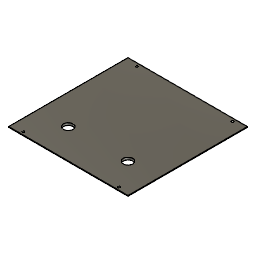
Sol 200x200mm (Autodesk Fusion 360 design; units mm, degrees)
part number: 2026-03-31-14-11-04-905
Autodesk Fusion 360 part; units mm, degrees
sketch "Esquisse1" plane through (0, 0, 0) normal (0, 0, 1) x (1, 0, 0)
  line L0 (0, 0) -> (200, 0)
  line L1 (200, 0) -> (200, 200)
  line L2 (200, 200) -> (0, 200)
  line L3 (0, 200) -> (0, 0)
  dimension "d18" = 200
  dimension "d19" = 200
  constraint horizontal L0
  constraint vertical L1
  constraint horizontal L2
  constraint vertical L3
  constraint coincident L0.start L3.end
  measures "d18" distance of L0 L2
  measures "d19" distance of L1 L3
extrude "Extrusion1" add sketch "Esquisse1" along normal blind 4
chamfer "Chanfrein1" distance 3 angle 45 1 faces at (66.6667, 133.3333, 0)
sketch "Esquisse2" plane through (0, 0, 4) normal (0, 0, 1) x (-1, 0, 0)
  circle A0 centre (-20, -195) radius 2
  circle A1 centre (-180, -195) radius 2
  circle A2 centre (-180, -5) radius 2
  circle A3 centre (-20, -5) radius 2
  line L0 (-20, -5) -> (-20, 0)
  line L1 (-180, -5) -> (-180, 0)
  line L2 (-20, -195) -> (-20, -200)
  line L3 (-180, -195) -> (-180, -200)
  line L4 (-20, -5) -> (0, -5)
  line L5 (-180, -5) -> (-200, -5)
  line L6 (-180, -195) -> (-200, -195)
  line L7 (-20, -195) -> (0, -195)
  line L8 (0, -200) -> (0, 0)
  line L9 (0, 0) -> (-200, 0)
  line L10 (-200, 0) -> (-200, -200)
  line L11 (-200, -200) -> (0, -200)
  dimension "d10" = 4
  dimension "d11" = 4
  dimension "d12" = 4
  dimension "d13" = 4
  dimension "d28" = 5
  dimension "d29" = 5
  dimension "d30" = 5
  dimension "d31" = 5
  dimension "d32" = 20
  dimension "d33" = 20
  dimension "d34" = 20
  dimension "d35" = 20
  constraint coincident A3.centre L0.start
  constraint coincident A2.centre L1.start
  constraint coincident A0.centre L2.start
  constraint coincident A1.centre L3.start
  measures "d10" diameter of A0
  measures "d11" diameter of A1
  measures "d12" diameter of A2
  measures "d13" diameter of A3
  measures "d28" distance of A3.centre L0.end
  measures "d29" distance of A2.centre L1.end
  measures "d30" distance of A0.centre L2.end
  measures "d31" distance of A1.centre L3.end
  measures "d32" distance of A3.centre L4.end
  measures "d33" distance of A2.centre L5.end
  measures "d34" distance of A0.centre L7.end
  measures "d35" distance of A1.centre L6.end
extrude "Extrusion2" cut sketch "Esquisse2" against normal blind 14 contours A0 L2 L7 | A0 L2 L7 | A3 L0 L4 | A3 L0 L4 | A1 L3 L6 | A1 L3 L6 | A2 L1 L5 | A2 L1 L5
thread "Filetage1" "ISO Metric profile 4.0 M4x0.7 M4x0.7 6H" major diameter 4.1095 minor diameter 3.332 pitch 0.7 angle 60 resizes the face on face at (20, 197, 2.6667)
thread "Filetage2" "ISO Metric profile 4.0 M4x0.7 M4x0.7 6H" major diameter 4.1095 minor diameter 3.332 pitch 0.7 angle 60 resizes the face on face at (20, 3, 2.6667)
thread "Filetage3" "ISO Metric profile 4.0 M4x0.7 M4x0.7 6H" major diameter 4.1095 minor diameter 3.332 pitch 0.7 angle 60 resizes the face on face at (180, 3, 2.6667)
thread "Filetage4" "ISO Metric profile 4.0 M4x0.7 M4x0.7 6H" major diameter 4.1095 minor diameter 3.332 pitch 0.7 angle 60 resizes the face on face at (180, 197, 2.6667)
move_face "DécalerLesFaces1" offset -0.05 1 faces at (18.3423, 5.1659, 2.6667)
move_face "DécalerLesFaces2" offset -0.05 1 faces at (180.5306, 6.5792, 2.6667)
move_face "DécalerLesFaces3" offset -0.05 1 faces at (178.3423, 195.1659, 1.3333)
move_face "DécalerLesFaces4" offset -0.05 1 faces at (18.3423, 195.1659, 2.6667)
sketch "Esquisse5" plane through (0, 0, 0) normal (0, 0, 1) x (1, 0, 0)
  line L0 (0, 49.9306) -> (50, 49.9306)
  line L1 (50, 0) -> (50, 50)
  circle A0 centre (50, 50) radius 8
  line L2 (150, 0) -> (150, 50)
  circle A1 centre (150, 50) radius 8
  line L3 (200, 49.9306) -> (150, 49.9306)
  dimension "d40" = 50
  dimension "d41" = 50
  dimension "d42" = 16
  dimension "d43" = 50
  dimension "d44" = 50
  dimension "d45" = 16
  constraint horizontal L0
  constraint vertical L1
  constraint coincident L1.end A0.centre
  measures "d40" distance of L0.start L0.end
  measures "d41" distance of L1.start L1.end
  measures "d42" diameter of A0
  measures "d43" distance of L3.end L3.start
  measures "d44" distance of L2.end L2.start
  measures "d45" diameter of A1
extrude "Extrusion3" cut sketch "Esquisse5" along normal blind 50
